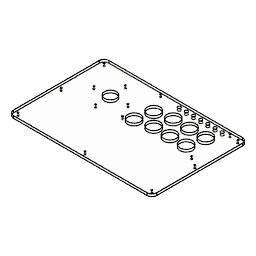
ArcadeStickAcrylicTopLayer (Autodesk Fusion 360 design; units mm, degrees)
part number: 2026-04-12-21-15-11-073
Autodesk Fusion 360 part; units mm, degrees
sketch "Sketch1" plane through (0, 0, 0) normal (0, 0, 1) x (1, 0, 0)
  line L0 (140, 100) -> (-140, 100)
  line L1 (-150, 90) -> (-150, -90)
  line L2 (-140, -100) -> (140, -100)
  line L3 (150, -90) -> (150, 90)
  line L4 (150, 100) -> (-150, -100) construction
  line L5 (-150, 100) -> (150, -100) construction
  arc A0 (-140, 100) -> (-150, 90) centre (-140, 90) ccw
  arc A1 (150, 90) -> (140, 100) centre (140, 90) ccw
  arc A2 (-150, -90) -> (-140, -100) centre (-140, -90) ccw
  arc A3 (140, -100) -> (150, -90) centre (140, -90) ccw
  circle A4 centre (-140, 90) radius 1.75
  circle A5 centre (-140, -90) radius 1.75
  circle A6 centre (140, -90) radius 1.75
  circle A7 centre (140, 90) radius 1.75
  circle A8 centre (-24.5, 93) radius 1.75
  circle A9 centre (120.5, 93) radius 1.75
  circle A10 centre (120.5, 13) radius 1.75
  circle A11 centre (-24.5, 13) radius 1.75
  circle A12 centre (-9.217, 22.009) radius 13.25
  circle A13 centre (-2.217, 56.009) radius 13.25
  circle A14 centre (24.783, 29.009) radius 13.25
  circle A15 centre (31.783, 63.009) radius 13.25
  circle A16 centre (65.783, 63.009) radius 13.25
  circle A17 centre (58.783, 29.009) radius 13.25
  circle A18 centre (92.783, 29.009) radius 13.25
  circle A19 centre (99.783, 63.009) radius 13.25
  circle A20 centre (108.5, 88.75) radius 3.25
  circle A21 centre (93.5, 88.75) radius 3.25
  circle A22 centre (78.5, 88.75) radius 3.25
  circle A23 centre (63.5, 88.75) radius 3.25
  circle A24 centre (33.5, 88.75) radius 3.25
  circle A25 centre (48.5, 88.75) radius 3.25
  circle A26 centre (18.5, 88.75) radius 3.25
  circle A27 centre (-75.717, 39.009) radius 12.5
  circle A28 centre (-77.417, 71.909) radius 1.75
  circle A29 centre (-108.617, 37.309) radius 1.75
  circle A30 centre (-74.017, 6.109) radius 1.75
  circle A31 centre (-40.817, 40.709) radius 1.75
  circle A32 centre (-140, 0) radius 1.75
  circle A33 centre (140, 0) radius 1.75
  circle A34 centre (0, -90) radius 1.75
  dimension "d1" = 300
  dimension "d2" = 200
  dimension "d3" = 10
  dimension "d4" = 10
  dimension "d5" = 10
  dimension "d6" = 10
  dimension "d7" = 3.5
  dimension "d8" = 3.5
  dimension "d9" = 3.5
  dimension "d10" = 3.5
  dimension "d13" = 3.5
  dimension "d14" = 145
  dimension "d15" = 3.5
  dimension "d16" = 3.5
  dimension "d17" = 145
  dimension "d18" = 3.5
  dimension "d21" = 26.5
  dimension "d22" = 26.5
  dimension "d23" = 26.5
  dimension "d24" = 26.5
  dimension "d25" = 26.5
  dimension "d26" = 26.5
  dimension "d27" = 26.5
  dimension "d28" = 26.5
  dimension "d31" = 6.5
  dimension "d32" = 6.5
  dimension "d33" = 6.5
  dimension "d34" = 6.5
  dimension "d35" = 6.5
  dimension "d36" = 6.5
  dimension "d37" = 6.5
  dimension "d41" = 25
  dimension "d44" = 3.5
  dimension "d58" = 3.5
  dimension "d59" = 3.5
  dimension "d60" = 3.5
  constraint horizontal L0
  constraint perpendicular L0 L1
  constraint parallel L0 L2
  constraint parallel L1 L3
  constraint coincident L4 origin
  constraint coincident L5 origin
  constraint coincident L5.start L0
  constraint coincident L5.start L1
  constraint tangent L0 A0
  constraint tangent L1 A0
  constraint coincident L4.start L0
  constraint coincident L4.start L3
  constraint tangent L0 A1
  constraint tangent L3 A1
  constraint coincident L4.end L1
  constraint coincident L4.end L2
  constraint tangent L1 A2
  constraint tangent L2 A2
  constraint coincident L5.end L3
  constraint coincident L5.end L2
  constraint tangent L3 A3
  constraint tangent L2 A3
  constraint concentric A0 A4
  constraint concentric A2 A5
  constraint concentric A3 A6
  constraint concentric A1 A7
  measures "d1" distance of L4.end L5.end
  measures "d2" distance of L5.start L4.end
  measures "d3" radius of A0
  measures "d4" radius of A1
  measures "d5" radius of A2
  measures "d6" radius of A3
  measures "d7" diameter of A4
  measures "d8" diameter of A5
  measures "d9" diameter of A6
  measures "d10" diameter of A7
  measures "d13" diameter of A8
  measures "d14" distance of A8.centre A9.centre
  measures "d15" diameter of A9
  measures "d16" diameter of A11
  measures "d17" distance of A11.centre A10.centre
  measures "d18" diameter of A10
  measures "d21" diameter of A12
  measures "d22" diameter of A13
  measures "d23" diameter of A14
  measures "d24" diameter of A15
  measures "d25" diameter of A17
  measures "d26" diameter of A16
  measures "d27" diameter of A18
  measures "d28" diameter of A19
  measures "d31" diameter of A20
  measures "d32" diameter of A21
  measures "d33" diameter of A22
  measures "d34" diameter of A23
  measures "d35" diameter of A25
  measures "d36" diameter of A24
  measures "d37" diameter of A26
  measures "d41" diameter of A27
  measures "d44" diameter of A28
  measures "d58" diameter of A32
  measures "d59" diameter of A33
  measures "d60" diameter of A34
sketch "Sketch2" plane through (0, 0, 5) normal (0, 0, 1) x (-1, 0, 0)
  circle A0 centre (77.417, -71.909) radius 1.75
  circle A1 centre (9.217, -22.009) radius 13.25
  circle A2 centre (-108.5, -88.75) radius 3.25
  circle A3 centre (-58.783, -29.009) radius 13.25
  circle A4 centre (-93.5, -88.75) radius 3.25
  circle A5 centre (40.817, -40.709) radius 1.75
  circle A6 centre (140, 90) radius 1.75
  circle A7 centre (24.5, -93) radius 1.75
  circle A8 centre (-63.5, -88.75) radius 3.25
  circle A9 centre (-18.5, -88.75) radius 3.25
  circle A10 centre (-99.783, -63.009) radius 13.25
  circle A11 centre (-33.5, -88.75) radius 3.25
  circle A12 centre (108.617, -37.309) radius 1.75
  circle A13 centre (-92.783, -29.009) radius 13.25
  circle A14 centre (-48.5, -88.75) radius 3.25
  circle A15 centre (-65.783, -63.009) radius 13.25
  circle A16 centre (140, -90) radius 1.75
  circle A17 centre (24.5, -13) radius 1.75
  circle A18 centre (-120.5, -13) radius 1.75
  circle A19 centre (-78.5, -88.75) radius 3.25
  circle A20 centre (-140, -90) radius 1.75
  circle A21 centre (-31.783, -63.009) radius 13.25
  circle A22 centre (-140, 90) radius 1.75
  circle A23 centre (74.017, -6.109) radius 1.75
  circle A24 centre (2.217, -56.009) radius 13.25
  circle A25 centre (75.717, -39.009) radius 12.5
  circle A26 centre (-120.5, -93) radius 1.75
  circle A27 centre (-24.783, -29.009) radius 13.25
  arc A28 (-140, 100) -> (-150, 90) centre (-140, 90) ccw
  line L0 (-150, 90) -> (-150, -90)
  arc A29 (-150, -90) -> (-140, -100) centre (-140, -90) ccw
  line L1 (-140, -100) -> (140, -100)
  arc A30 (140, -100) -> (150, -90) centre (140, -90) ccw
  line L2 (150, -90) -> (150, 90)
  arc A31 (150, 90) -> (140, 100) centre (140, 90) ccw
  line L3 (140, 100) -> (-140, 100)
  circle A32 centre (77.717, -62.659) radius 1.75
  circle A33 centre (99.367, -37.009) radius 1.75
  circle A34 centre (73.717, -15.359) radius 1.75
  circle A35 centre (52.067, -41.009) radius 1.75
  dimension "d53" = 3.5
  dimension "d55" = 360
  measures "d53" diameter of A32
extrude "Extrude4" add sketch "Sketch1" along normal blind 5
extrude "Extrude5" cut sketch "Sketch2" against normal blind 5 contours A32 | A33 | A34 | A35
sketch "Sketch3" plane through (0, 0, 5) normal (0, 0, 1) x (-1, 0, 0)
  circle A0 centre (99.367, -37.009) radius 1.75
  circle A1 centre (73.717, -15.359) radius 1.75
  circle A2 centre (77.717, -62.659) radius 1.75
  circle A3 centre (52.067, -41.009) radius 1.75
  circle A4 centre (140, 0) radius 1.75
  circle A5 centre (-63.5, -88.75) radius 3.25
  circle A6 centre (108.617, -37.309) radius 1.75
  circle A7 centre (-140, 0) radius 1.75
  circle A8 centre (-48.5, -88.75) radius 3.25
  circle A9 centre (-108.5, -88.75) radius 3.25
  circle A10 centre (24.5, -13) radius 1.75
  circle A11 centre (-78.5, -88.75) radius 3.25
  circle A12 centre (9.217, -22.009) radius 13.25
  circle A13 centre (-140, -90) radius 1.75
  circle A14 centre (2.217, -56.009) radius 13.25
  circle A15 centre (-120.5, -13) radius 1.75
  circle A16 centre (-120.5, -93) radius 1.75
  circle A17 centre (-31.783, -63.009) radius 13.25
  circle A18 centre (140, 90) radius 1.75
  circle A19 centre (75.717, -39.009) radius 12.5
  circle A20 centre (-18.5, -88.75) radius 3.25
  circle A21 centre (-58.783, -29.009) radius 13.25
  circle A22 centre (-65.783, -63.009) radius 13.25
  circle A23 centre (40.817, -40.709) radius 1.75
  circle A24 centre (24.5, -93) radius 1.75
  circle A25 centre (-140, 90) radius 1.75
  circle A26 centre (-99.783, -63.009) radius 13.25
  circle A27 centre (-92.783, -29.009) radius 13.25
  circle A28 centre (140, -90) radius 1.75
  circle A29 centre (77.417, -71.909) radius 1.75
  circle A30 centre (74.017, -6.109) radius 1.75
  circle A31 centre (-24.783, -29.009) radius 13.25
  circle A32 centre (0, 90) radius 1.75
  circle A33 centre (-33.5, -88.75) radius 3.25
  circle A34 centre (-93.5, -88.75) radius 3.25
  arc A35 (-140, 100) -> (-150, 90) centre (-140, 90) ccw
  line L0 (-150, 90) -> (-150, -90)
  arc A36 (-150, -90) -> (-140, -100) centre (-140, -90) ccw
  line L1 (-140, -100) -> (140, -100)
  arc A37 (140, -100) -> (150, -90) centre (140, -90) ccw
  line L2 (150, -90) -> (150, 90)
  arc A38 (150, 90) -> (140, 100) centre (140, 90) ccw
  line L3 (140, 100) -> (-140, 100)
extrude "Extrude6" add sketch "Sketch2" against normal up to surface (5 mm away) contours A32 | A33 | A34 | A35
extrude "Extrude1" [suppressed]
